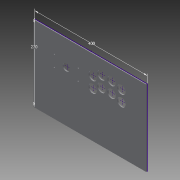
# Autodesk Inventor part: Panel_top_2
Saved by Autodesk Inventor 2013 (Build 170138000, 138)
## iProperties
Created: 2013-01-09
Part Number: Panel_top_2
Material: Generic
Document SubType Name: Modeling
Designer: mstine
Density: 1 g/cm^3
Author: mstine
Autodesk Inventor part; units mm, degrees
ref_plane "YZ Plane" through (0, 0, 0) normal (1, 0, 0) x (0, 1, 0)
ref_plane "XZ Plane" through (0, 0, 0) normal (0, 1, 0) x (-1, 0, 0)
ref_plane "XY Plane" through (0, 0, 0) normal (0, 0, 1) x (1, 0, 0)
sketch "Panel" plane through (0, 0, 0) normal (0, 0, 1) x (1, 0, 0)
  line L0 (-200, 135) -> (200, 135)
  line L1 (200, 135) -> (200, -135)
  line L2 (200, -135) -> (-200, -135)
  line L3 (-200, -135) -> (-200, 135)
  point P0 (0, 0)
  point P1 (-200, 0)
  point P2 (0, 135)
  dimension "d0" = 270
  dimension "d3" = 400
  constraints: 8 end point, 2 midpoint, 2 parallel, 1 horizontal, 1 horizontal alignment, 1 perpendicular, 1 vertical alignment
  measures "d0" distance of L2.end L0.start
  measures "d3" distance of L0.start L0.end
sketch "JoystickMount" plane through (0, 0, 0) normal (0, 0, 1) x (1, 0, 0)
  line L0 (-127.5, 65.25) -> (-127.5, 24.75) construction
  line L1 (-127.5, 24.75) -> (-42.5, 24.75) construction
  point P0 (0, 0)
  point P1 (-85, 45)
  point P2 (-42.5, 65.25)
  point P3 (-127.5, 45)
  point P4 (-85, 24.75)
  dimension "d4" = 40.5
  dimension "d6" = 85
  dimension "d19" = 45
  dimension "d45" = 85
  constraints: 4 end point, 3 horizontal alignment, 3 vertical alignment, 2 midpoint, 1 perpendicular, 1 vertical
  measures "d4" distance of L0.start L0.end
  measures "d6" distance of L0.end L1.end
  measures "d19" vertical distance of point (0, 0) point (-85, 45)
  measures "d45" horizontal distance of point (0, 0) point (-85, 45)
sketch "ButtonMounts" plane through (0, 0, 0) normal (0, 0, 1) x (1, 0, 0)
  point P0 (0, 0)
  point P1 (10, 66)
  point P2 (10, 27)
  point P3 (41.25, 84)
  point P4 (41.25, 45)
  point P5 (77.25, 84)
  point P6 (77.25, 45)
  point P7 (112.25, 75)
  point P8 (112.25, 36)
  point P9 (-85, 45)
  dimension "d7" = 39
  dimension "d9" = 39
  dimension "d10" = 39
  dimension "d11" = 39
  dimension "d12" = 31.25
  dimension "d13" = 36
  dimension "d14" = 35
  dimension "d15" = 18
  dimension "d16" = 9
  dimension "d17" = 95
  constraints: 4 vertical alignment, 2 horizontal alignment
  measures "d7" distance of point (10, 27) point (10, 66)
  measures "d9" distance of point (41.25, 84) point (41.25, 45)
  measures "d10" distance of point (77.25, 45) point (77.25, 84)
  measures "d11" distance of point (112.25, 36) point (112.25, 75)
  measures "d12" horizontal distance of point (41.25, 45) point (10, 27)
  measures "d13" distance of point (41.25, 45) point (77.25, 45)
  measures "d14" horizontal distance of point (77.25, 45) point (112.25, 36)
  measures "d15" vertical distance of point (10, 27) point (41.25, 45)
  measures "d16" vertical distance of point (112.25, 36) point (77.25, 45)
  measures "d17" horizontal distance of point (10, 27) point (-85, 45)
extrude "PanelExtrusion" add sketch "Panel" along normal blind 4
hole "JoystickScrews" at (-42.5, 24.75, 0) at (-42.5, 65.25, 0) at (-127.5, 65.25, 0) at (-127.5, 24.75, 0) direction (0, 0, 1) diameter 5 end through all
hole "JoystickShaft" at (-85, 45, 0) direction (0, 0, 1) diameter 24 end through all
hole "ButtonHoles" at (112.25, 36, 0) at (77.25, 45, 0) at (77.25, 84, 0) at (112.25, 75, 0) at (41.25, 84, 0) at (41.25, 45, 0) at (10, 66, 0) at (10, 27, 0) direction (0, 0, 1) diameter 30 end through all
body "Solid2"
